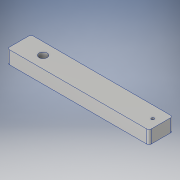
# Autodesk Inventor part: Transmisor_grande
Saved by Autodesk Inventor 2019 (Build 230136000, 136)
## iProperties
Created: 2019-09-30
Part Number: Transmisor_grande
Material: Aluminum 6061
Document SubType Name: Modeling
Designer: Domenico
Density: 2.7 g/cm^3
Appearance: Aluminum - Flat
Mass: 426.013 g
Surface Area: 284.517 cm^2
Volume: 157.783 cm^3
Diametro_eje_pequeño: 4.000 mm
ancho: 32.700 mm
separacion_grande: 33.000 mm
Author: Domenico
Autodesk Inventor part; units mm, degrees
ref_plane "YZ Plane" through (0, 0, 0) normal (1, 0, 0) x (0, 1, 0)
ref_plane "XZ Plane" through (0, 0, 0) normal (0, 1, 0) x (-1, 0, 0)
ref_plane "XY Plane" through (0, 0, 0) normal (0, 0, 1) x (1, 0, 0)
sketch "Sketch1" plane through (0, 0, 0) normal (0, 1, 0) x (-1, 0, 0)
  line L0 (0, 0) -> (-195, 0)
  line L1 (-195, 0) -> (-195, -32.7)
  line L2 (-195, -32.7) -> (0, -32.7)
  line L3 (0, -32.7) -> (0, 0)
  circle A0 centre (-33, -16.35) radius 5.5563
  circle A1 centre (-183.8875, -16.35) radius 2
  point P0 (0, -16.35)
  point P1 (-195, -16.35)
  dimension "d0" = 195
  dimension "ancho" = 32.7
  dimension "separacion_grande" = 33
  dimension "d3" = 11.1125
  dimension "d4" = 11.1125
  dimension "Diametro_eje_pequeño" = 4
  constraints: 8 end point, 2 centre point, 2 horizontal alignment, 2 midpoint, 2 parallel, 1 horizontal, 1 perpendicular
  measures "d0" distance of L2.end L1.end
  measures "ancho" distance of L0.end L1.end
  measures "separacion_grande" distance from line of L3 A0.centre
  measures "d3" diameter of A0
  measures "d4" distance from line of L1 A1.centre
  measures "Diametro_eje_pequeño" diameter of A1
extrude "Extrusion1" add sketch "Sketch1" along normal blind 18
fillet "Fillet1" radius 3 4 edges at (0, 9, 0) (195, 9, 0) (195, 9, -32.7) (0, 9, -32.7)
equation "\"d3\" = diametro_interno"
equation "\"d4\" = d3"
equation "\"diametro_interno\" = 11.1125"
body "Solid1"
